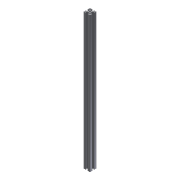
# Autodesk Inventor part: KHFS5-2020-4000
Saved by Autodesk Inventor 2014 SP1 (Build 180222100, 222)
## iProperties
Category: PARTsolutions
Created: 2015-02-04
Part Number: KHFS5-2020-4000
Catalog Web Link: www.cadenas.de
Description: KHFS5-2020-4000, KHFSB5-2020-4000, KHFSF5-2020-4000, KHFSFB5-2020-4000, KHFST5-2020-4000, KHFSTB5-2020-4000, KHFSH5-2020-4000, KHFSC5-2020-4000 - HFS5 Series Aluminum Extrusions 20,25,40mm Square -1 Slot-
Document SubType Name: Modeling
Designer: PARTsolutions
Material: Generic
Density: 1 g/cm^3
Appearance: RGB(175,175,175)
NB: KHFS5-2020-4000
NN: KHFS5-2020-4000, KHFSB5-2020-4000, KHFSF5-2020-4000, KHFSFB5-2020-4000, KHFST5-2020-4000, KHFSTB5-2020-4000, KHFSH5-2020-4000, KHFSC5-2020-4000
NT: HFS5 Series Aluminum Extrusions 20,25,40mm Square -1 Slot-
NBSYN: $PN.
LINA: KHFS5-2020-4000
PN: KHFS5-2020-4000
TPS: KHFS5-2020
TP: KHFS5
FRM: 2020
MAT: A6N01SS-T5 Aluminum Alloy or 6005A-T5 Aluminum Alloy
ST: Clear Anodize
FEAT: Four-Side Slots
L: 4000
LTOL: +/- 0.5
MASS: 0
SA: 183
GMILX: 0.742x10^4
GMILY: 0.742x10^4
CLF: HFS5-2020
WIDTH: 20.000
HEIGHT: 20.000
VER: 1
DIM: 1
DRILLDIA: 4.200
KT: 1
CreationOption_UseAsmMates: 0
SUPPLIER: Misumi
ARTICLENO: KHFS5-2020-4000
BOMINFO: KHFS5-2020-4000
CREATOR: CADENAS GmbH
PSOL_IDENT_0: {\\10.0.0.236\data_v8\23d-libs\misumi\metric\38_al_extrusions_blackets\5\khfs5_2020.prj},309 {VTYP=3
PSOL_IDENT_1: D},{NB=KHFS5-2020-4000},{LINA=KHFS5-2020-4000},{NN=KHFS5-2020-4000, KHFSB5-2020-4000, KHFSF5-2020-40
PSOL_IDENT_2: 00, KHFSFB5-2020-4000, KHFST5-2020-4000, KHFSTB5-2020-4000, KHFSH5-2020-4000, KHFSC5-2020-4000},{DAT
PSOL_IDENT_3: E=19.11.2014 02:28:13},{GEOMDATE=07.04.2011 07:46:00},{VERSION=},{LINEID=10},{LINESUBID=-1},{WBVAR=}
PSOL_IDENT_4: {NB=KHFS5-2020-4000},{LINA=KHFS5-2020-4000},{KT=1},{PN=KHFS5-2020-4000},{TPS=KHFS5-2020},{TP=KHFS5
PSOL_IDENT_5: },{FRM=2020},{MAT=A6N01SS-T5 Aluminum Alloy or 6005A-T5 Aluminum Alloy},{ST=Clear Anodize},{FEAT=Fou
PSOL_IDENT_6: r-Side Slots},{L=4000},{LTOL=+/- 0.5},{MASS=0},{SA=183},{GMILX=0.742x10^4},{GMILY=0.742x10^4},{CLF=H
PSOL_IDENT_7: FS5-2020},{WIDTH=20.000},{HEIGHT=20.000},{VER=1},{DIM=1},{DRILLDIA=4.200}
Title: KHFS5-2020-4000
Author: Cadenas PARTsolutions
Comments: HFS5 Series Aluminum Extrusions 20,25,40mm Square -1 Slot-
Autodesk Inventor part; units mm, degrees
ref_plane "YZ Plane" through (0, 0, 0) normal (1, 0, 0) x (0, 1, 0)
ref_plane "XZ Plane" through (0, 0, 0) normal (0, 1, 0) x (-1, 0, 0)
ref_plane "XY Plane" through (0, 0, 0) normal (0, 0, 1) x (1, 0, 0)
sketch "Sketch_5" plane through (0, 0, 0) normal (0, 0, 1) x (1, 0, 0)
  line L0 (-10, 9) -> (-10, 3.3)
  arc A0 (-10, 3.3) -> (-9.7, 3) centre (-9.7, 3.3) ccw
  line L1 (-9.7, 3) -> (-8, 3)
  line L2 (-8, 3) -> (-8, 6)
  line L3 (-8, 6) -> (-7.0607, 6)
  line L4 (-7.0607, 6) -> (-4, 2.9393)
  line L5 (-4, 2.9393) -> (-4, 0.3)
  line L6 (-4, 0.3) -> (-3.7, 0)
  line L7 (-3.7, 0) -> (-4, -0.3)
  line L8 (-4, -0.3) -> (-4, -2.9393)
  line L9 (-4, -2.9393) -> (-7.0607, -6)
  line L10 (-7.0607, -6) -> (-8, -6)
  line L11 (-8, -6) -> (-8, -3)
  line L12 (-8, -3) -> (-9.7, -3)
  arc A1 (-9.7, -3) -> (-10, -3.3) centre (-9.7, -3.3) ccw
  line L13 (-10, -3.3) -> (-10, -9)
  arc A2 (-10, -9) -> (-9, -10) centre (-9, -9) ccw
  line L14 (-9, -10) -> (-3.3, -10)
  arc A3 (-3.3, -10) -> (-3, -9.7) centre (-3.3, -9.7) ccw
  line L15 (-3, -9.7) -> (-3, -8)
  line L16 (-3, -8) -> (-6, -8)
  line L17 (-6, -8) -> (-6, -7.0607)
  line L18 (-6, -7.0607) -> (-2.9393, -4)
  line L19 (-2.9393, -4) -> (-0.3, -4)
  line L20 (-0.3, -4) -> (0, -3.7)
  line L21 (0, -3.7) -> (0.3, -4)
  line L22 (0.3, -4) -> (2.9393, -4)
  line L23 (2.9393, -4) -> (6, -7.0607)
  line L24 (6, -7.0607) -> (6, -8)
  line L25 (6, -8) -> (3, -8)
  line L26 (3, -8) -> (3, -9.7)
  arc A4 (3, -9.7) -> (3.3, -10) centre (3.3, -9.7) ccw
  line L27 (3.3, -10) -> (9, -10)
  arc A5 (9, -10) -> (10, -9) centre (9, -9) ccw
  line L28 (10, -9) -> (10, -3.3)
  arc A6 (10, -3.3) -> (9.7, -3) centre (9.7, -3.3) ccw
  line L29 (9.7, -3) -> (8, -3)
  line L30 (8, -3) -> (8, -6)
  line L31 (8, -6) -> (7.0607, -6)
  line L32 (7.0607, -6) -> (4, -2.9393)
  line L33 (4, -2.9393) -> (4, -0.3)
  line L34 (4, -0.3) -> (3.7, 0)
  line L35 (3.7, 0) -> (4, 0.3)
  line L36 (4, 0.3) -> (4, 2.9393)
  line L37 (4, 2.9393) -> (7.0607, 6)
  line L38 (7.0607, 6) -> (8, 6)
  line L39 (8, 6) -> (8, 3)
  line L40 (8, 3) -> (9.7, 3)
  arc A7 (9.7, 3) -> (10, 3.3) centre (9.7, 3.3) ccw
  line L41 (10, 3.3) -> (10, 9)
  arc A8 (10, 9) -> (9, 10) centre (9, 9) ccw
  line L42 (9, 10) -> (3.3, 10)
  arc A9 (3.3, 10) -> (3, 9.7) centre (3.3, 9.7) ccw
  line L43 (3, 9.7) -> (3, 8)
  line L44 (3, 8) -> (6, 8)
  line L45 (6, 8) -> (6, 7.0607)
  line L46 (6, 7.0607) -> (2.9393, 4)
  line L47 (2.9393, 4) -> (0.3, 4)
  line L48 (0.3, 4) -> (0, 3.7)
  line L49 (0, 3.7) -> (-0.3, 4)
  line L50 (-0.3, 4) -> (-2.9393, 4)
  line L51 (-2.9393, 4) -> (-6, 7.0607)
  line L52 (-6, 7.0607) -> (-6, 8)
  line L53 (-6, 8) -> (-3, 8)
  line L54 (-3, 8) -> (-3, 9.7)
  arc A10 (-3, 9.7) -> (-3.3, 10) centre (-3.3, 9.7) ccw
  line L55 (-3.3, 10) -> (-9, 10)
  arc A11 (-9, 10) -> (-10, 9) centre (-9, 9) ccw
  circle A12 centre (0, 0) radius 2.1
  constraints: 112 end point, 24 point on circle, 13 centre point
extrude "Extrusion1" add sketch "Sketch_5" against normal blind 426
body "Solid1"
